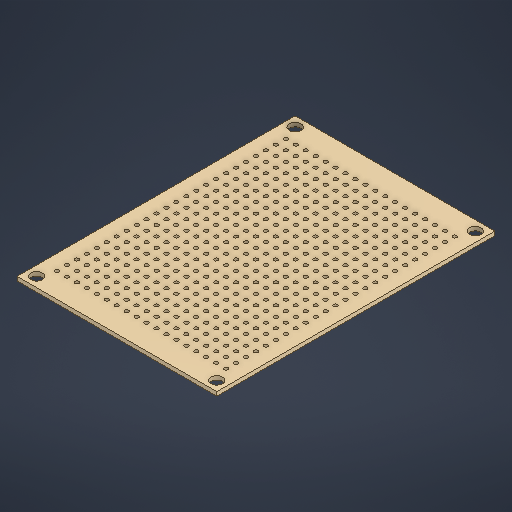
# Autodesk Inventor part: perfboard-71x51x1
Saved by Autodesk Inventor 2025.2 (Build 292293000, 293)
## iProperties
Created: 2025-11-15
Part Number: perfboard-71x51x1
Material: Fiberglass Batt
Document SubType Name: Modeling
Designer: sam
Density: 0.032 g/cm^3
Appearance: Golden Sand
Author: sam
Autodesk Inventor part; units mm, degrees
ref_plane "YZ Plane" through (0, 0, 0) normal (1, 0, 0) x (0, 1, 0)
ref_plane "XZ Plane" through (0, 0, 0) normal (0, 1, 0) x (-1, 0, 0)
ref_plane "XY Plane" through (0, 0, 0) normal (0, 0, 1) x (1, 0, 0)
sketch "Sketch1" plane through (0, 0, 0) normal (0, 1, 0) x (-1, 0, 0)
  line L0 (-25.5, -35.5) -> (25.5, -35.5)
  line L1 (25.5, -35.5) -> (25.5, 35.5)
  line L2 (25.5, 35.5) -> (-25.5, 35.5)
  line L3 (-25.5, 35.5) -> (-25.5, -35.5)
  line L4 (-25.5, -35.5) -> (25.5, 35.5) construction
  line L5 (25.5, -35.5) -> (-25.5, 35.5) construction
  circle A0 centre (21.59, -29.21) radius 0.5
  circle A1 centre (19.05, -29.21) radius 0.5
  circle A2 centre (16.51, -29.21) radius 0.5
  circle A3 centre (13.97, -29.21) radius 0.5
  circle A4 centre (11.43, -29.21) radius 0.5
  circle A5 centre (8.89, -29.21) radius 0.5
  circle A6 centre (6.35, -29.21) radius 0.5
  circle A7 centre (3.81, -29.21) radius 0.5
  circle A8 centre (1.27, -29.21) radius 0.5
  circle A9 centre (-1.27, -29.21) radius 0.5
  circle A10 centre (-3.81, -29.21) radius 0.5
  circle A11 centre (-6.35, -29.21) radius 0.5
  circle A12 centre (-8.89, -29.21) radius 0.5
  circle A13 centre (-11.43, -29.21) radius 0.5
  circle A14 centre (-13.97, -29.21) radius 0.5
  circle A15 centre (-16.51, -29.21) radius 0.5
  circle A16 centre (-19.05, -29.21) radius 0.5
  circle A17 centre (-21.59, -29.21) radius 0.5
  circle A18 centre (21.59, -26.67) radius 0.5
  circle A19 centre (19.05, -26.67) radius 0.5
  circle A20 centre (16.51, -26.67) radius 0.5
  circle A21 centre (13.97, -26.67) radius 0.5
  circle A22 centre (11.43, -26.67) radius 0.5
  circle A23 centre (8.89, -26.67) radius 0.5
  circle A24 centre (6.35, -26.67) radius 0.5
  circle A25 centre (3.81, -26.67) radius 0.5
  circle A26 centre (1.27, -26.67) radius 0.5
  circle A27 centre (-1.27, -26.67) radius 0.5
  circle A28 centre (-3.81, -26.67) radius 0.5
  circle A29 centre (-6.35, -26.67) radius 0.5
  circle A30 centre (-8.89, -26.67) radius 0.5
  circle A31 centre (-11.43, -26.67) radius 0.5
  circle A32 centre (-13.97, -26.67) radius 0.5
  circle A33 centre (-16.51, -26.67) radius 0.5
  circle A34 centre (-19.05, -26.67) radius 0.5
  circle A35 centre (-21.59, -26.67) radius 0.5
  circle A36 centre (21.59, -24.13) radius 0.5
  circle A37 centre (19.05, -24.13) radius 0.5
  circle A38 centre (16.51, -24.13) radius 0.5
  circle A39 centre (13.97, -24.13) radius 0.5
  circle A40 centre (11.43, -24.13) radius 0.5
  circle A41 centre (8.89, -24.13) radius 0.5
  circle A42 centre (6.35, -24.13) radius 0.5
  circle A43 centre (3.81, -24.13) radius 0.5
  circle A44 centre (1.27, -24.13) radius 0.5
  circle A45 centre (-1.27, -24.13) radius 0.5
  circle A46 centre (-3.81, -24.13) radius 0.5
  circle A47 centre (-6.35, -24.13) radius 0.5
  circle A48 centre (-8.89, -24.13) radius 0.5
  circle A49 centre (-11.43, -24.13) radius 0.5
  circle A50 centre (-13.97, -24.13) radius 0.5
  circle A51 centre (-16.51, -24.13) radius 0.5
  circle A52 centre (-19.05, -24.13) radius 0.5
  circle A53 centre (-21.59, -24.13) radius 0.5
  circle A54 centre (21.59, -21.59) radius 0.5
  circle A55 centre (19.05, -21.59) radius 0.5
  circle A56 centre (16.51, -21.59) radius 0.5
  circle A57 centre (13.97, -21.59) radius 0.5
  circle A58 centre (11.43, -21.59) radius 0.5
  circle A59 centre (8.89, -21.59) radius 0.5
  circle A60 centre (6.35, -21.59) radius 0.5
  circle A61 centre (3.81, -21.59) radius 0.5
  circle A62 centre (1.27, -21.59) radius 0.5
  circle A63 centre (-1.27, -21.59) radius 0.5
  circle A64 centre (-3.81, -21.59) radius 0.5
  circle A65 centre (-6.35, -21.59) radius 0.5
  circle A66 centre (-8.89, -21.59) radius 0.5
  circle A67 centre (-11.43, -21.59) radius 0.5
  circle A68 centre (-13.97, -21.59) radius 0.5
  circle A69 centre (-16.51, -21.59) radius 0.5
  circle A70 centre (-19.05, -21.59) radius 0.5
  circle A71 centre (-21.59, -21.59) radius 0.5
  circle A72 centre (21.59, -19.05) radius 0.5
  circle A73 centre (19.05, -19.05) radius 0.5
  circle A74 centre (16.51, -19.05) radius 0.5
  circle A75 centre (13.97, -19.05) radius 0.5
  circle A76 centre (11.43, -19.05) radius 0.5
  circle A77 centre (8.89, -19.05) radius 0.5
  circle A78 centre (6.35, -19.05) radius 0.5
  circle A79 centre (3.81, -19.05) radius 0.5
  circle A80 centre (1.27, -19.05) radius 0.5
  circle A81 centre (-1.27, -19.05) radius 0.5
  circle A82 centre (-3.81, -19.05) radius 0.5
  circle A83 centre (-6.35, -19.05) radius 0.5
  circle A84 centre (-8.89, -19.05) radius 0.5
  circle A85 centre (-11.43, -19.05) radius 0.5
  circle A86 centre (-13.97, -19.05) radius 0.5
  circle A87 centre (-16.51, -19.05) radius 0.5
  circle A88 centre (-19.05, -19.05) radius 0.5
  circle A89 centre (-21.59, -19.05) radius 0.5
  circle A90 centre (21.59, -16.51) radius 0.5
  circle A91 centre (19.05, -16.51) radius 0.5
  circle A92 centre (16.51, -16.51) radius 0.5
  circle A93 centre (13.97, -16.51) radius 0.5
  circle A94 centre (11.43, -16.51) radius 0.5
  circle A95 centre (8.89, -16.51) radius 0.5
  circle A96 centre (6.35, -16.51) radius 0.5
  circle A97 centre (3.81, -16.51) radius 0.5
  circle A98 centre (1.27, -16.51) radius 0.5
  circle A99 centre (-1.27, -16.51) radius 0.5
  circle A100 centre (-3.81, -16.51) radius 0.5
  circle A101 centre (-6.35, -16.51) radius 0.5
  circle A102 centre (-8.89, -16.51) radius 0.5
  circle A103 centre (-11.43, -16.51) radius 0.5
  circle A104 centre (-13.97, -16.51) radius 0.5
  circle A105 centre (-16.51, -16.51) radius 0.5
  circle A106 centre (-19.05, -16.51) radius 0.5
  circle A107 centre (-21.59, -16.51) radius 0.5
  circle A108 centre (21.59, -13.97) radius 0.5
  circle A109 centre (19.05, -13.97) radius 0.5
  circle A110 centre (16.51, -13.97) radius 0.5
  circle A111 centre (13.97, -13.97) radius 0.5
  circle A112 centre (11.43, -13.97) radius 0.5
  circle A113 centre (8.89, -13.97) radius 0.5
  circle A114 centre (6.35, -13.97) radius 0.5
  circle A115 centre (3.81, -13.97) radius 0.5
  circle A116 centre (1.27, -13.97) radius 0.5
  circle A117 centre (-1.27, -13.97) radius 0.5
  circle A118 centre (-3.81, -13.97) radius 0.5
  circle A119 centre (-6.35, -13.97) radius 0.5
  circle A120 centre (-8.89, -13.97) radius 0.5
  circle A121 centre (-11.43, -13.97) radius 0.5
  circle A122 centre (-13.97, -13.97) radius 0.5
  circle A123 centre (-16.51, -13.97) radius 0.5
  circle A124 centre (-19.05, -13.97) radius 0.5
  circle A125 centre (-21.59, -13.97) radius 0.5
  circle A126 centre (21.59, -11.43) radius 0.5
  circle A127 centre (19.05, -11.43) radius 0.5
  circle A128 centre (16.51, -11.43) radius 0.5
  circle A129 centre (13.97, -11.43) radius 0.5
  circle A130 centre (11.43, -11.43) radius 0.5
  circle A131 centre (8.89, -11.43) radius 0.5
  circle A132 centre (6.35, -11.43) radius 0.5
  circle A133 centre (3.81, -11.43) radius 0.5
  circle A134 centre (1.27, -11.43) radius 0.5
  circle A135 centre (-1.27, -11.43) radius 0.5
  circle A136 centre (-3.81, -11.43) radius 0.5
  circle A137 centre (-6.35, -11.43) radius 0.5
  circle A138 centre (-8.89, -11.43) radius 0.5
  circle A139 centre (-11.43, -11.43) radius 0.5
  circle A140 centre (-13.97, -11.43) radius 0.5
  circle A141 centre (-16.51, -11.43) radius 0.5
  circle A142 centre (-19.05, -11.43) radius 0.5
  circle A143 centre (-21.59, -11.43) radius 0.5
  circle A144 centre (21.59, -8.89) radius 0.5
  circle A145 centre (19.05, -8.89) radius 0.5
  circle A146 centre (16.51, -8.89) radius 0.5
  circle A147 centre (13.97, -8.89) radius 0.5
  circle A148 centre (11.43, -8.89) radius 0.5
  circle A149 centre (8.89, -8.89) radius 0.5
  circle A150 centre (6.35, -8.89) radius 0.5
  circle A151 centre (3.81, -8.89) radius 0.5
  circle A152 centre (1.27, -8.89) radius 0.5
  circle A153 centre (-1.27, -8.89) radius 0.5
  circle A154 centre (-3.81, -8.89) radius 0.5
  circle A155 centre (-6.35, -8.89) radius 0.5
  circle A156 centre (-8.89, -8.89) radius 0.5
  circle A157 centre (-11.43, -8.89) radius 0.5
  circle A158 centre (-13.97, -8.89) radius 0.5
  circle A159 centre (-16.51, -8.89) radius 0.5
  circle A160 centre (-19.05, -8.89) radius 0.5
  circle A161 centre (-21.59, -8.89) radius 0.5
  circle A162 centre (21.59, -6.35) radius 0.5
  circle A163 centre (19.05, -6.35) radius 0.5
  circle A164 centre (16.51, -6.35) radius 0.5
  circle A165 centre (13.97, -6.35) radius 0.5
  circle A166 centre (11.43, -6.35) radius 0.5
  circle A167 centre (8.89, -6.35) radius 0.5
  circle A168 centre (6.35, -6.35) radius 0.5
  circle A169 centre (3.81, -6.35) radius 0.5
  circle A170 centre (1.27, -6.35) radius 0.5
  circle A171 centre (-1.27, -6.35) radius 0.5
  circle A172 centre (-3.81, -6.35) radius 0.5
  circle A173 centre (-6.35, -6.35) radius 0.5
  circle A174 centre (-8.89, -6.35) radius 0.5
  circle A175 centre (-11.43, -6.35) radius 0.5
  circle A176 centre (-13.97, -6.35) radius 0.5
  circle A177 centre (-16.51, -6.35) radius 0.5
  circle A178 centre (-19.05, -6.35) radius 0.5
  circle A179 centre (-21.59, -6.35) radius 0.5
  circle A180 centre (21.59, -3.81) radius 0.5
  circle A181 centre (19.05, -3.81) radius 0.5
  circle A182 centre (16.51, -3.81) radius 0.5
  circle A183 centre (13.97, -3.81) radius 0.5
  circle A184 centre (11.43, -3.81) radius 0.5
  circle A185 centre (8.89, -3.81) radius 0.5
  circle A186 centre (6.35, -3.81) radius 0.5
  circle A187 centre (3.81, -3.81) radius 0.5
  circle A188 centre (1.27, -3.81) radius 0.5
  circle A189 centre (-1.27, -3.81) radius 0.5
  circle A190 centre (-3.81, -3.81) radius 0.5
  circle A191 centre (-6.35, -3.81) radius 0.5
  circle A192 centre (-8.89, -3.81) radius 0.5
  circle A193 centre (-11.43, -3.81) radius 0.5
  circle A194 centre (-13.97, -3.81) radius 0.5
  circle A195 centre (-16.51, -3.81) radius 0.5
  circle A196 centre (-19.05, -3.81) radius 0.5
  circle A197 centre (-21.59, -3.81) radius 0.5
  circle A198 centre (21.59, -1.27) radius 0.5
  circle A199 centre (19.05, -1.27) radius 0.5
  circle A200 centre (16.51, -1.27) radius 0.5
  circle A201 centre (13.97, -1.27) radius 0.5
  circle A202 centre (11.43, -1.27) radius 0.5
  circle A203 centre (8.89, -1.27) radius 0.5
  circle A204 centre (6.35, -1.27) radius 0.5
  circle A205 centre (3.81, -1.27) radius 0.5
  circle A206 centre (1.27, -1.27) radius 0.5
  circle A207 centre (-1.27, -1.27) radius 0.5
  circle A208 centre (-3.81, -1.27) radius 0.5
  circle A209 centre (-6.35, -1.27) radius 0.5
  circle A210 centre (-8.89, -1.27) radius 0.5
  circle A211 centre (-11.43, -1.27) radius 0.5
  circle A212 centre (-13.97, -1.27) radius 0.5
  circle A213 centre (-16.51, -1.27) radius 0.5
  circle A214 centre (-19.05, -1.27) radius 0.5
  circle A215 centre (-21.59, -1.27) radius 0.5
  circle A216 centre (21.59, 1.27) radius 0.5
  circle A217 centre (19.05, 1.27) radius 0.5
  circle A218 centre (16.51, 1.27) radius 0.5
  circle A219 centre (13.97, 1.27) radius 0.5
  circle A220 centre (11.43, 1.27) radius 0.5
  circle A221 centre (8.89, 1.27) radius 0.5
  circle A222 centre (6.35, 1.27) radius 0.5
  circle A223 centre (3.81, 1.27) radius 0.5
  circle A224 centre (1.27, 1.27) radius 0.5
  circle A225 centre (-1.27, 1.27) radius 0.5
  circle A226 centre (-3.81, 1.27) radius 0.5
  circle A227 centre (-6.35, 1.27) radius 0.5
  circle A228 centre (-8.89, 1.27) radius 0.5
  circle A229 centre (-11.43, 1.27) radius 0.5
  circle A230 centre (-13.97, 1.27) radius 0.5
  circle A231 centre (-16.51, 1.27) radius 0.5
  circle A232 centre (-19.05, 1.27) radius 0.5
  circle A233 centre (-21.59, 1.27) radius 0.5
  circle A234 centre (21.59, 3.81) radius 0.5
  circle A235 centre (19.05, 3.81) radius 0.5
  circle A236 centre (16.51, 3.81) radius 0.5
  circle A237 centre (13.97, 3.81) radius 0.5
  circle A238 centre (11.43, 3.81) radius 0.5
  circle A239 centre (8.89, 3.81) radius 0.5
  circle A240 centre (6.35, 3.81) radius 0.5
  circle A241 centre (3.81, 3.81) radius 0.5
  circle A242 centre (1.27, 3.81) radius 0.5
  circle A243 centre (-1.27, 3.81) radius 0.5
  circle A244 centre (-3.81, 3.81) radius 0.5
  circle A245 centre (-6.35, 3.81) radius 0.5
  circle A246 centre (-8.89, 3.81) radius 0.5
  circle A247 centre (-11.43, 3.81) radius 0.5
  circle A248 centre (-13.97, 3.81) radius 0.5
  circle A249 centre (-16.51, 3.81) radius 0.5
  circle A250 centre (-19.05, 3.81) radius 0.5
  circle A251 centre (-21.59, 3.81) radius 0.5
  circle A252 centre (21.59, 6.35) radius 0.5
  circle A253 centre (19.05, 6.35) radius 0.5
  circle A254 centre (16.51, 6.35) radius 0.5
  circle A255 centre (13.97, 6.35) radius 0.5
  circle A256 centre (11.43, 6.35) radius 0.5
  circle A257 centre (8.89, 6.35) radius 0.5
  circle A258 centre (6.35, 6.35) radius 0.5
  circle A259 centre (3.81, 6.35) radius 0.5
  circle A260 centre (1.27, 6.35) radius 0.5
  circle A261 centre (-1.27, 6.35) radius 0.5
  circle A262 centre (-3.81, 6.35) radius 0.5
  circle A263 centre (-6.35, 6.35) radius 0.5
  circle A264 centre (-8.89, 6.35) radius 0.5
  circle A265 centre (-11.43, 6.35) radius 0.5
  circle A266 centre (-13.97, 6.35) radius 0.5
  circle A267 centre (-16.51, 6.35) radius 0.5
  circle A268 centre (-19.05, 6.35) radius 0.5
  circle A269 centre (-21.59, 6.35) radius 0.5
  circle A270 centre (21.59, 8.89) radius 0.5
  circle A271 centre (19.05, 8.89) radius 0.5
  circle A272 centre (16.51, 8.89) radius 0.5
  circle A273 centre (13.97, 8.89) radius 0.5
  circle A274 centre (11.43, 8.89) radius 0.5
  circle A275 centre (8.89, 8.89) radius 0.5
  circle A276 centre (6.35, 8.89) radius 0.5
  circle A277 centre (3.81, 8.89) radius 0.5
  circle A278 centre (1.27, 8.89) radius 0.5
  circle A279 centre (-1.27, 8.89) radius 0.5
  circle A280 centre (-3.81, 8.89) radius 0.5
  circle A281 centre (-6.35, 8.89) radius 0.5
  circle A282 centre (-8.89, 8.89) radius 0.5
  circle A283 centre (-11.43, 8.89) radius 0.5
  circle A284 centre (-13.97, 8.89) radius 0.5
  circle A285 centre (-16.51, 8.89) radius 0.5
  circle A286 centre (-19.05, 8.89) radius 0.5
  circle A287 centre (-21.59, 8.89) radius 0.5
  circle A288 centre (21.59, 11.43) radius 0.5
  circle A289 centre (19.05, 11.43) radius 0.5
  circle A290 centre (16.51, 11.43) radius 0.5
  circle A291 centre (13.97, 11.43) radius 0.5
  circle A292 centre (11.43, 11.43) radius 0.5
  circle A293 centre (8.89, 11.43) radius 0.5
  circle A294 centre (6.35, 11.43) radius 0.5
  circle A295 centre (3.81, 11.43) radius 0.5
  circle A296 centre (1.27, 11.43) radius 0.5
  circle A297 centre (-1.27, 11.43) radius 0.5
  circle A298 centre (-3.81, 11.43) radius 0.5
  circle A299 centre (-6.35, 11.43) radius 0.5
  circle A300 centre (-8.89, 11.43) radius 0.5
  circle A301 centre (-11.43, 11.43) radius 0.5
  circle A302 centre (-13.97, 11.43) radius 0.5
  circle A303 centre (-16.51, 11.43) radius 0.5
  circle A304 centre (-19.05, 11.43) radius 0.5
  circle A305 centre (-21.59, 11.43) radius 0.5
  circle A306 centre (21.59, 13.97) radius 0.5
  circle A307 centre (19.05, 13.97) radius 0.5
  circle A308 centre (16.51, 13.97) radius 0.5
  circle A309 centre (13.97, 13.97) radius 0.5
  circle A310 centre (11.43, 13.97) radius 0.5
  circle A311 centre (8.89, 13.97) radius 0.5
  circle A312 centre (6.35, 13.97) radius 0.5
  circle A313 centre (3.81, 13.97) radius 0.5
  circle A314 centre (1.27, 13.97) radius 0.5
  circle A315 centre (-1.27, 13.97) radius 0.5
  circle A316 centre (-3.81, 13.97) radius 0.5
  circle A317 centre (-6.35, 13.97) radius 0.5
  circle A318 centre (-8.89, 13.97) radius 0.5
  circle A319 centre (-11.43, 13.97) radius 0.5
  circle A320 centre (-13.97, 13.97) radius 0.5
  circle A321 centre (-16.51, 13.97) radius 0.5
  circle A322 centre (-19.05, 13.97) radius 0.5
  circle A323 centre (-21.59, 13.97) radius 0.5
  circle A324 centre (21.59, 16.51) radius 0.5
  circle A325 centre (19.05, 16.51) radius 0.5
  circle A326 centre (16.51, 16.51) radius 0.5
  circle A327 centre (13.97, 16.51) radius 0.5
  circle A328 centre (11.43, 16.51) radius 0.5
  circle A329 centre (8.89, 16.51) radius 0.5
  circle A330 centre (6.35, 16.51) radius 0.5
  circle A331 centre (3.81, 16.51) radius 0.5
  circle A332 centre (1.27, 16.51) radius 0.5
  circle A333 centre (-1.27, 16.51) radius 0.5
  circle A334 centre (-3.81, 16.51) radius 0.5
  circle A335 centre (-6.35, 16.51) radius 0.5
  circle A336 centre (-8.89, 16.51) radius 0.5
  circle A337 centre (-11.43, 16.51) radius 0.5
  circle A338 centre (-13.97, 16.51) radius 0.5
  circle A339 centre (-16.51, 16.51) radius 0.5
  circle A340 centre (-19.05, 16.51) radius 0.5
  circle A341 centre (-21.59, 16.51) radius 0.5
  circle A342 centre (21.59, 19.05) radius 0.5
  circle A343 centre (19.05, 19.05) radius 0.5
  circle A344 centre (16.51, 19.05) radius 0.5
  circle A345 centre (13.97, 19.05) radius 0.5
  circle A346 centre (11.43, 19.05) radius 0.5
  circle A347 centre (8.89, 19.05) radius 0.5
  circle A348 centre (6.35, 19.05) radius 0.5
  circle A349 centre (3.81, 19.05) radius 0.5
  circle A350 centre (1.27, 19.05) radius 0.5
  circle A351 centre (-1.27, 19.05) radius 0.5
  circle A352 centre (-3.81, 19.05) radius 0.5
  circle A353 centre (-6.35, 19.05) radius 0.5
  circle A354 centre (-8.89, 19.05) radius 0.5
  circle A355 centre (-11.43, 19.05) radius 0.5
  circle A356 centre (-13.97, 19.05) radius 0.5
  circle A357 centre (-16.51, 19.05) radius 0.5
  circle A358 centre (-19.05, 19.05) radius 0.5
  circle A359 centre (-21.59, 19.05) radius 0.5
  circle A360 centre (21.59, 21.59) radius 0.5
  circle A361 centre (19.05, 21.59) radius 0.5
  circle A362 centre (16.51, 21.59) radius 0.5
  circle A363 centre (13.97, 21.59) radius 0.5
  circle A364 centre (11.43, 21.59) radius 0.5
  circle A365 centre (8.89, 21.59) radius 0.5
  circle A366 centre (6.35, 21.59) radius 0.5
  circle A367 centre (3.81, 21.59) radius 0.5
  circle A368 centre (1.27, 21.59) radius 0.5
  circle A369 centre (-1.27, 21.59) radius 0.5
  circle A370 centre (-3.81, 21.59) radius 0.5
  circle A371 centre (-6.35, 21.59) radius 0.5
  circle A372 centre (-8.89, 21.59) radius 0.5
  circle A373 centre (-11.43, 21.59) radius 0.5
  circle A374 centre (-13.97, 21.59) radius 0.5
  circle A375 centre (-16.51, 21.59) radius 0.5
  circle A376 centre (-19.05, 21.59) radius 0.5
  circle A377 centre (-21.59, 21.59) radius 0.5
  circle A378 centre (21.59, 24.13) radius 0.5
  circle A379 centre (19.05, 24.13) radius 0.5
  circle A380 centre (16.51, 24.13) radius 0.5
  circle A381 centre (13.97, 24.13) radius 0.5
  circle A382 centre (11.43, 24.13) radius 0.5
  circle A383 centre (8.89, 24.13) radius 0.5
  circle A384 centre (6.35, 24.13) radius 0.5
  circle A385 centre (3.81, 24.13) radius 0.5
  circle A386 centre (1.27, 24.13) radius 0.5
  circle A387 centre (-1.27, 24.13) radius 0.5
  circle A388 centre (-3.81, 24.13) radius 0.5
  circle A389 centre (-6.35, 24.13) radius 0.5
  circle A390 centre (-8.89, 24.13) radius 0.5
  circle A391 centre (-11.43, 24.13) radius 0.5
  circle A392 centre (-13.97, 24.13) radius 0.5
  circle A393 centre (-16.51, 24.13) radius 0.5
  circle A394 centre (-19.05, 24.13) radius 0.5
  circle A395 centre (-21.59, 24.13) radius 0.5
  circle A396 centre (21.59, 26.67) radius 0.5
  circle A397 centre (19.05, 26.67) radius 0.5
  circle A398 centre (16.51, 26.67) radius 0.5
  circle A399 centre (13.97, 26.67) radius 0.5
  circle A400 centre (11.43, 26.67) radius 0.5
  circle A401 centre (8.89, 26.67) radius 0.5
  circle A402 centre (6.35, 26.67) radius 0.5
  circle A403 centre (3.81, 26.67) radius 0.5
  circle A404 centre (1.27, 26.67) radius 0.5
  circle A405 centre (-1.27, 26.67) radius 0.5
  circle A406 centre (-3.81, 26.67) radius 0.5
  circle A407 centre (-6.35, 26.67) radius 0.5
  circle A408 centre (-8.89, 26.67) radius 0.5
  circle A409 centre (-11.43, 26.67) radius 0.5
  circle A410 centre (-13.97, 26.67) radius 0.5
  circle A411 centre (-16.51, 26.67) radius 0.5
  circle A412 centre (-19.05, 26.67) radius 0.5
  circle A413 centre (-21.59, 26.67) radius 0.5
  circle A414 centre (21.59, 29.21) radius 0.5
  circle A415 centre (19.05, 29.21) radius 0.5
  circle A416 centre (16.51, 29.21) radius 0.5
  circle A417 centre (13.97, 29.21) radius 0.5
  circle A418 centre (11.43, 29.21) radius 0.5
  circle A419 centre (8.89, 29.21) radius 0.5
  circle A420 centre (6.35, 29.21) radius 0.5
  circle A421 centre (3.81, 29.21) radius 0.5
  circle A422 centre (1.27, 29.21) radius 0.5
  circle A423 centre (-1.27, 29.21) radius 0.5
  circle A424 centre (-3.81, 29.21) radius 0.5
  circle A425 centre (-6.35, 29.21) radius 0.5
  circle A426 centre (-8.89, 29.21) radius 0.5
  circle A427 centre (-11.43, 29.21) radius 0.5
  circle A428 centre (-13.97, 29.21) radius 0.5
  circle A429 centre (-16.51, 29.21) radius 0.5
  circle A430 centre (-19.05, 29.21) radius 0.5
  circle A431 centre (-21.59, 29.21) radius 0.5
  circle A432 centre (-23, -33) radius 1.5
  circle A433 centre (-23, 33) radius 1.5
  circle A434 centre (23, 33) radius 1.5
  circle A435 centre (23, -33) radius 1.5
  point P0 (0, 0)
  dimension "d0" = 51
  dimension "d1" = 71
  dimension "d2" = 1
  dimension "d5" = 2.54
  dimension "d8" = 2.54
  dimension "d11" = 6.29
  dimension "d12" = 3.91
  dimension "d13" = 3
  dimension "d14" = 2.5
  dimension "d15" = 2.5
  dimension "d16" = 3
  dimension "d17" = 2.5
  dimension "d18" = 2.5
  dimension "d19" = 3
  dimension "d20" = 2.5
  dimension "d21" = 2.5
  dimension "d22" = 3
  dimension "d23" = 2.5
  dimension "d24" = 2.5
  constraints: 436 centre point, 12 end point, 2 horizontal, 2 midpoint, 2 parallel, 1 perpendicular, 1 vertical, 862 other
  measures "d0" distance of L2.end L1.end
  measures "d1" distance of L1.end L0.end
  measures "d2" diameter of A0
  measures "d5" distance of A0.centre A1.centre
  measures "d8" distance of A0.centre A18.centre
  measures "d11" distance from line of L0 A0.centre
  measures "d12" distance from line of L1 A0.centre
  measures "d13" diameter of A432
  measures "d14" distance from line of L0 A432.centre
  measures "d15" distance from line of L3 A432.centre
  measures "d16" diameter of A433
  measures "d17" distance from line of L3 A433.centre
  measures "d18" distance from line of L2 A433.centre
  measures "d19" diameter of A434
  measures "d20" distance from line of L2 A434.centre
  measures "d21" distance from line of L1 A434.centre
  measures "d22" diameter of A435
  measures "d23" distance from line of L1 A435.centre
  measures "d24" distance from line of L0 A435.centre
extrude "Extrusion1" add sketch "Sketch1" along normal blind 1
body "Solid1"
